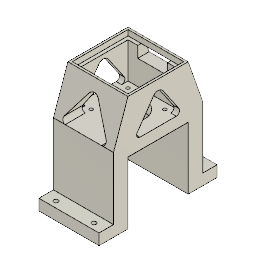
Motor Holder v19 (Autodesk Fusion 360 design; units mm, degrees)
Autodesk Fusion 360 part; units mm, degrees
sketch "Sketch1" plane through (0, 0, 0) normal (0, 0, 1) x (1, 0, 0)
  circle A0 centre (16.5, 16.5) radius 1.5
  circle A1 centre (16.5, -16.5) radius 1.5
  circle A2 centre (-16.5, -16.5) radius 1.5
  circle A3 centre (-16.5, 16.5) radius 1.5
  circle A4 centre (0, 0) radius 15
  line L0 (27, 27) -> (-27, 27)
  line L1 (-27, 27) -> (-27, -27)
  line L2 (-27, -27) -> (27, -27)
  line L3 (27, -27) -> (27, 27)
  line L4 (27, 27) -> (-27, -27) construction
  line L5 (-27, 27) -> (27, -27) construction
  dimension "d1" = 33
  dimension "d2" = 33
  dimension "d3" = 3
  dimension "d4" = 3
  dimension "d5" = 3
  dimension "d6" = 3
  dimension "d7" = 30
  dimension "d8" = 54
  dimension "d9" = 54
  constraint coincident A4.centre origin
  constraint perpendicular L0 L1
  constraint parallel L0 L2
  constraint parallel L1 L3
  constraint horizontal L0
  constraint coincident L4 A4.centre
  constraint coincident L5 A4.centre
  measures "d1" distance of A1.centre A2.centre
  measures "d2" distance of A2.centre A3.centre
  measures "d3" diameter of A0
  measures "d4" diameter of A1
  measures "d5" diameter of A2
  measures "d6" diameter of A3
  measures "d7" diameter of A4
  measures "d8" distance of L1.end L2.end
  measures "d9" distance of L0.end L1.end
extrude "Extrude1" add sketch "Sketch1" along normal blind 5 makes body 1
sketch "Sketch2" plane through (0, 0, 5) normal (0, 0, 1) x (-1, 0, 0)
  circle A0 centre (0, 0) radius 15
  circle A1 centre (-16.5, -16.5) radius 1.5
  circle A2 centre (16.5, -16.5) radius 1.5
  circle A3 centre (16.5, 16.5) radius 1.5
  circle A4 centre (-16.5, 16.5) radius 1.5
  line L0 (-27, 27) -> (-27, -27)
  line L1 (-27, -27) -> (27, -27)
  line L2 (27, -27) -> (27, 27)
  line L3 (27, 27) -> (-27, 27)
  line L4 (-22, -22) -> (22, -22)
  line L5 (22, -22) -> (22, 22)
  line L6 (22, 22) -> (-22, 22)
  line L7 (-22, 22) -> (-22, -22)
  line L8 (-22, -22) -> (22, 22) construction
  line L9 (22, -22) -> (-22, 22) construction
  dimension "d12" = 44
  dimension "d13" = 44
  constraint perpendicular L4 L5
  constraint parallel L4 L6
  constraint parallel L5 L7
  constraint horizontal L4
  constraint coincident L8 A0.centre
  constraint coincident L9 A0.centre
  constraint coincident A0.centre origin
  measures "d12" distance of L5.end L6.end
  measures "d13" distance of L4.end L5.end
extrude "Extrude2" add sketch "Sketch2" along normal blind 37 contours L0 L1 L2 L3 bodies 1
sketch "Sketch3" plane through (0, 0, 42) normal (0, 0, 1) x (-1, 0, 0)
  line L0 (-22, -22) -> (-22, 22)
  line L1 (-22, 22) -> (22, 22)
  line L2 (22, 22) -> (22, -22)
  line L3 (22, -22) -> (-22, -22)
  line L4 (27, 27) -> (-27, 27)
  line L5 (-27, 27) -> (-27, -27)
  line L6 (-27, -27) -> (27, -27)
  line L7 (27, -27) -> (27, 27)
  line L8 (-25, -25) -> (25, -25)
  line L9 (25, -25) -> (25, 25)
  line L10 (25, 25) -> (-25, 25)
  line L11 (-25, 25) -> (-25, -25)
  line L12 (-25, -25) -> (25, 25) construction
  line L13 (25, -25) -> (-25, 25) construction
  constraint perpendicular L8 L9
  constraint parallel L8 L10
  constraint parallel L9 L11
  constraint horizontal L8
  constraint coincident L12 origin
  constraint coincident L13 origin
extrude "Extrude3" cut sketch "Sketch3" against normal blind 5 contours L8 L9 L10 L11 bodies 1
sketch "Sketch4" plane through (0, 0, 0) normal (0, 0, -1) x (1, 0, 0)
  circle A0 centre (0, 0) radius 15
  circle A1 centre (16.5, -16.5) radius 1.5
  circle A2 centre (-16.5, -16.5) radius 1.5
  circle A3 centre (-16.5, 16.5) radius 1.5
  circle A4 centre (16.5, 16.5) radius 1.5
  line L0 (27, -27) -> (27, 27)
  line L1 (27, 27) -> (-27, 27)
  line L2 (-27, 27) -> (-27, -27)
  line L3 (-27, -27) -> (27, -27)
sketch "Sketch5" plane through (0, 0, 0) normal (0, 0, -1) x (1, 0, 0)
sketch "Sketch6" plane through (0, 0, 5) normal (0, 0, 1) x (-1, 0, 0)
  line L0 (-22, -22) -> (22, -22)
  line L1 (22, -22) -> (22, 22)
  line L2 (22, 22) -> (-22, 22)
  line L3 (-22, 22) -> (-22, -22)
  circle A0 centre (0, 0) radius 15
  circle A1 centre (-16.5, -16.5) radius 1.5
  circle A2 centre (16.5, -16.5) radius 1.5
  circle A3 centre (16.5, 16.5) radius 1.5
  circle A4 centre (-16.5, 16.5) radius 1.5
  line L4 (-27, -40) -> (27, -40)
  line L5 (27, -40) -> (27, 40)
  line L6 (27, 40) -> (-27, 40)
  line L7 (-27, 40) -> (-27, -40)
  line L8 (-27, -40) -> (27, 40) construction
  line L9 (27, -40) -> (-27, 40) construction
  circle A5 centre (16.5, 16.5) radius 1.5
  circle A6 centre (0, 0) radius 15
  circle A7 centre (-16.5, 16.5) radius 1.5
  circle A8 centre (-16.5, -16.5) radius 1.5
  circle A9 centre (16.5, -16.5) radius 1.5
  dimension "d18" = 80
  constraint perpendicular L4 L5
  constraint parallel L4 L6
  constraint parallel L5 L7
  constraint horizontal L4
  constraint coincident L8 A0.centre
  constraint coincident L9 A0.centre
  constraint coincident A0.centre A6.centre
  constraint concentric A3 A5
  constraint concentric A4 A7
  constraint concentric A1 A8
  constraint concentric A2 A9
  measures "d18" distance of L4.end L5.end
extrude "Extrude4" add sketch "Sketch6" against normal blind 10 contours L4 L5 L6 L7 bodies 1
extrude "Extrude5" add sketch "Sketch4" along normal blind 5 bodies 1
sketch "Sketch7" plane through (0, 0, -5) normal (0, 0, -1) x (1, 0, 0)
  circle A0 centre (-16.5, 16.5) radius 1.5
  circle A1 centre (16.5, 16.5) radius 1.5
  circle A2 centre (0, 0) radius 15
  circle A3 centre (-16.5, -16.5) radius 1.5
  circle A4 centre (16.5, -16.5) radius 1.5
  line L0 (27, -40) -> (27, 40)
  line L1 (27, 40) -> (-27, 40)
  line L2 (-27, 40) -> (-27, -40)
  line L3 (-27, -40) -> (27, -40)
  line L4 (27, -40) -> (-27, -40)
  line L5 (-27, -40) -> (-27, -27)
  line L6 (-27, -27) -> (27, -27)
  line L7 (27, -27) -> (27, -40)
  line L8 (27, 40) -> (-27, 40)
  line L9 (-27, 40) -> (-27, 27)
  line L10 (-27, 27) -> (27, 27)
  line L11 (27, 27) -> (27, 40)
  dimension "d23" = 13
  dimension "d24" = 13
  constraint horizontal L4
  constraint vertical L5
  constraint horizontal L6
  constraint vertical L7
  constraint coincident L0.start L3.end
  constraint horizontal L8
  constraint vertical L9
  constraint horizontal L10
  constraint vertical L11
  constraint coincident L0.end L1.start
  measures "d23" distance of L0.start L6.end
  measures "d24" distance of L0.end L10.end
extrude "Extrude6" add sketch "Sketch7" along normal blind 46 contours L0 L2 L3 L4 L5 L6 L7 | L0 L1 L2 L8 L9 L10 L11 bodies 1
sketch "Sketch8" plane through (0, 0, -51) normal (0, 0, -1) x (1, 0, 0)
  line L0 (27, 27) -> (27, 40)
  line L1 (27, 40) -> (-27, 40)
  line L2 (-27, 40) -> (-27, 27)
  line L3 (-27, 27) -> (27, 27)
  line L4 (27, 27) -> (-27, 27)
  line L5 (-27, 27) -> (-27, 53)
  line L6 (-27, 53) -> (27, 53)
  line L7 (27, 53) -> (27, 27)
  line L8 (27, -27) -> (-27, -27)
  line L9 (-27, -27) -> (-27, -53)
  line L10 (-27, -53) -> (27, -53)
  line L11 (27, -53) -> (27, -27)
  line L12 (27, 53) -> (27, 47.5)
  circle A0 centre (17.0346, 47.5) radius 2
  line L13 (0, 53) -> (0, 40)
  line L14 (27, 0) -> (15, 0)
  circle A1 centre (-17.0346, 47.5) radius 2
  circle A2 centre (17.0346, -47.5) radius 2
  circle A3 centre (-17.0346, -47.5) radius 2
  dimension "d27" = 5.5
  dimension "d28" = 4
  constraint horizontal L4
  constraint vertical L5
  constraint horizontal L6
  constraint vertical L7
  constraint coincident L0.start L3.end
  constraint horizontal L8
  constraint vertical L9
  constraint horizontal L10
  constraint vertical L11
  constraint perpendicular L1 L12
  constraint midpoint L6 L13.start
  constraint midpoint L1 L13.end
  constraint perpendicular L1 L13
  constraint perpendicular L13 L14
  constraint symmetric A0 L13 A1
  constraint symmetric A0 L14 A2
  constraint symmetric L14 A1 A3
  measures "d27" distance of L6.end L12.end
  measures "d28" diameter of A0
extrude "Extrude7" add sketch "Sketch8" along normal blind 10 bodies 1
sketch "Sketch9" plane through (-27, 0, 0) normal (-1, 0, 0) x (0, -1, 0)
  line L0 (40, -51) -> (40, 5)
  line L1 (40, 5) -> (27, 5)
  line L2 (27, 5) -> (27, 42)
  line L3 (27, 42) -> (-27, 42)
  line L4 (-27, 42) -> (-27, 5)
  line L5 (-27, 5) -> (-40, 5)
  line L6 (-40, 5) -> (-40, -51)
  line L7 (-40, -51) -> (-53, -51)
  line L8 (-53, -51) -> (-53, -61)
  line L9 (-53, -61) -> (-27, -61)
  line L10 (-27, -61) -> (-27, -5)
  line L11 (-27, -5) -> (27, -5)
  line L12 (27, -5) -> (27, -61)
  line L13 (27, -61) -> (53, -61)
  line L14 (53, -61) -> (53, -51)
  line L15 (53, -51) -> (40, -51)
  line L16 (-27, 42) -> (-40, 5)
  line L17 (-40, 5) -> (-53, -51)
  line L18 (27, 42) -> (40, 5)
  line L19 (40, 5) -> (53, -51)
  constraint coincident L3.end L4.start
  constraint coincident L5.end L6.start
  constraint coincident L7.end L8.start
  constraint coincident L2.end L3.start
  constraint coincident L0.end L1.start
  constraint coincident L14.end L15.start
extrude "Extrude8" add sketch "Sketch9" against normal blind 54 contours L1 L2 L18 | L4 L5 L16 bodies 1
sketch "Sketch10" plane through (22, 0, 0) normal (-1, 0, 0) x (0, -1, 0)
  line L0 (22, 37) -> (-22, 37)
  line L1 (-22, 37) -> (-22, 5)
  line L2 (-22, 5) -> (22, 5)
  line L3 (22, 5) -> (22, 37)
  line L4 (-18.769, 9.6996) -> (-4.1202, 31.007)
  line L5 (4.1202, 31.007) -> (18.769, 9.6996)
  line L6 (16.2969, 5) -> (-16.2969, 5)
  arc A0 (4.1202, 31.007) -> (-4.1202, 31.007) centre (0, 28.1743) ccw
  arc A1 (-18.769, 9.6996) -> (-16.2969, 5) centre (-16.2969, 8) ccw
  arc A2 (16.2969, 5) -> (18.769, 9.6996) centre (16.2969, 8) ccw
  dimension "d33" = 5
  dimension "d34" = 3
  dimension "d35" = 3
  constraint tangent L4 A0
  constraint tangent L5 A0
  constraint tangent L4 A1
  constraint tangent L6 A1
  constraint tangent L5 A2
  constraint tangent L6 A2
  measures "d33" radius of A0
  measures "d34" radius of A1
  measures "d35" radius of A2
extrude "Extrude9" cut sketch "Sketch10" along normal through all and the other way through all contours L2 L4 L5 L6 A0 A1 A2 bodies 1
sketch "Sketch11" plane through (0, -22, 0) normal (0, 1, 0) x (-1, 0, 0)
  line L0 (22, 37) -> (-22, 37)
  line L1 (-22, 37) -> (-22, 5)
  line L2 (-22, 5) -> (22, 5)
  line L3 (22, 5) -> (22, 37)
  line L4 (-18.769, 9.6996) -> (-4.1202, 31.007)
  line L5 (4.1202, 31.007) -> (18.769, 9.6996)
  line L6 (16.2969, 5) -> (-16.2969, 5)
  arc A0 (4.1202, 31.007) -> (-4.1202, 31.007) centre (0, 28.1743) ccw
  arc A1 (-18.769, 9.6996) -> (-16.2969, 5) centre (-16.2969, 8) ccw
  arc A2 (16.2969, 5) -> (18.769, 9.6996) centre (16.2969, 8) ccw
  dimension "d38" = 5
  dimension "d39" = 3
  dimension "d40" = 3
  constraint tangent L4 A0
  constraint tangent L5 A0
  constraint tangent L4 A1
  constraint tangent L6 A1
  constraint tangent L5 A2
  constraint tangent L6 A2
  measures "d38" radius of A0
  measures "d39" radius of A1
  measures "d40" radius of A2
extrude "Extrude10" cut sketch "Sketch11" against normal blind 30 contours L2 L4 L5 L6 A0 A1 A2 bodies 1
sketch "Sketch12" plane through (0, 22, 0) normal (0, -1, 0) x (1, 0, 0)
  line L0 (22, 37) -> (-22, 37)
  line L1 (-22, 37) -> (-22, 5)
  line L2 (-22, 5) -> (22, 5)
  line L3 (22, 5) -> (22, 37)
  line L4 (13.2773, 37) -> (-13.2773, 37)
  line L5 (-13.2773, 37) -> (-13.2773, 27)
  line L6 (-13.2773, 27) -> (13.2773, 27)
  line L7 (13.2773, 27) -> (13.2773, 37)
  line L8 (13.2773, 37) -> (-13.2773, 27) construction
  line L9 (-13.2773, 37) -> (13.2773, 27) construction
  point P0 (0, 32)
  constraint perpendicular L4 L5
  constraint parallel L4 L6
  constraint parallel L5 L7
  constraint horizontal L4
  constraint coincident L0 L4.start
  constraint coincident L8 P0
  constraint coincident L9 P0
extrude "Extrude11" cut sketch "Sketch12" against normal blind 12 contours L0 L4 L5 L6 L7 bodies 1
imported_body "Base Feature1" makes body 2 in component "Lower Parts"
move_body "Move1" [suppressed] in component "Lower Parts"
delete_face "DeleteFace1" [suppressed]
delete_face "DeleteFace2" [suppressed]
sketch "Sketch13" plane through (45, 0, 0) normal (1, 0, 0) x (0, 1, 0)
  line L0 (42, -49) -> (46, -49)
  line L1 (46, -49) -> (46, 8)
  line L2 (46, 8) -> (42, 8)
  line L3 (42, 8) -> (42, -49)
  line L4 (42, -49) -> (40, -49)
  line L5 (40, -49) -> (40, -51)
  line L6 (40, -51) -> (42, -51)
  line L7 (42, -51) -> (42, -49)
  constraint horizontal L4
  constraint vertical L5
  constraint horizontal L6
  constraint vertical L7
  constraint coincident L0.start L3.end
extrude "Extrude1'" [suppressed] in component "Lower Parts"
sketch "Sketch14" plane through (0, 42, 0) normal (0, 1, 0) x (-1, 0, 0)
  line L0 (-43, -51) -> (-45, -49)
  line L1 (-45, -49) -> (-45, -51)
  line L2 (-45, -51) -> (-43, -51)
  line L3 (-45, -49) -> (-43, -51)
  line L4 (-45, -49) -> (-45, -51)
  line L5 (-45, -51) -> (-43, -51)
  constraint coincident L0.end L1.start
  constraint coincident L0.start L2.end
  constraint coincident L1.end L2.start
extrude "Extrude2'" [suppressed] in component "Lower Parts"
extrude "Extrude3'" [suppressed] in component "Lower Parts"
extrude "Extrude4'" [suppressed] in component "Lower Parts"
combine "Combine1" [suppressed]
extrude "Extrude12" [suppressed]
sketch "Sketch15" plane through (0, 0, -51) normal (0, 0, 1) x (-1, 0, 0)
  line L0 (27, -46) -> (-27, -46)
  line L1 (-27, -46) -> (-27, -68)
  line L2 (-27, -68) -> (27, -68)
  line L3 (27, -68) -> (27, -46)
  point P0 (13, -57)
  point P1 (-13, -57)
hole "Hole1" [suppressed]
delete_face "DeleteFace3" [suppressed]
delete_face "DeleteFace4" [suppressed]
extrude "Extrude13" [suppressed]
fillet "Fillet1" [suppressed]
sketch "Sketch16" plane through (0, 0, -51) normal (0, 0, 1) x (-1, 0, 0)
  line L0 (-27, 48.5) -> (27, 48.5)
  line L1 (27, 48.5) -> (27, 63)
  line L2 (27, 63) -> (-27, 63)
  line L3 (-27, 63) -> (-27, 48.5)
  point P0 (13, 54)
  point P1 (-13, 54)
hole "Hole2" [suppressed]
sketch "Sketch17" plane through (0, 27, 0) normal (0, -1, 0) x (1, 0, 0)
  line L0 (27, -5) -> (-27, -5)
  line L1 (-27, -5) -> (-27, -61)
  line L2 (-27, -61) -> (27, -61)
  line L3 (27, -61) -> (27, -5)
  line L4 (0, -61) -> (-4, -61)
  line L5 (-4, -61) -> (-4, -51)
  circle A0 centre (-4, -42.5) radius 8.5
  constraint midpoint L2 L4.start
  constraint coincident L2 L4.end
  constraint parallel L2 L4
  constraint perpendicular L0 L5
  constraint coincident L5.end A0
extrude "Extrude14" [suppressed]
component "Lower Parts" placed x (-1, 0, 0) y (0, 1, 0) z (0, 0, -1) at (-16, 41.7309, -23.7483)
named bodies: "L Body"
